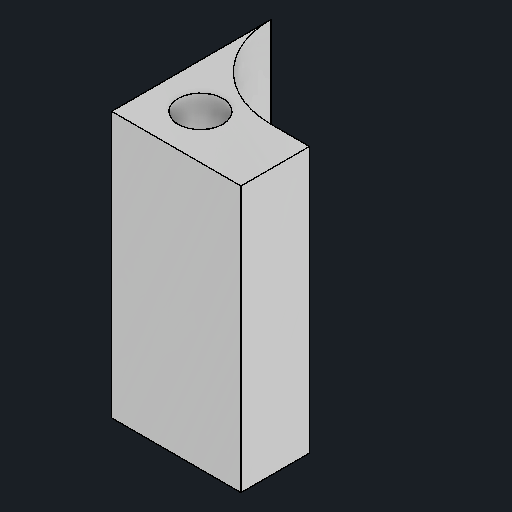
# Autodesk Inventor part: Joint Spacer
Saved by Autodesk Inventor 2026.1 (Build 301233020, 233B)
## iProperties
Created: 2025-05-26
Part Number: Joint Spacer
Material: Aluminum 6061
Document SubType Name: Modeling
Designer: Joshua Eah
Density: 2.7 g/cm^3
Appearance: Machined - Aluminum
Author: Joshua Eah
Autodesk Inventor part; units mm, degrees
ref_plane "YZ Plane" through (0, 0, 0) normal (1, 0, 0) x (0, 1, 0)
ref_plane "XZ Plane" through (0, 0, 0) normal (0, 1, 0) x (-1, 0, 0)
ref_plane "XY Plane" through (0, 0, 0) normal (0, 0, 1) x (1, 0, 0)
sketch "Base" plane through (0, 0, 0) normal (0, 1, 0) x (-1, 0, 0)
  line L0 (0, 0) -> (-12, 0)
  line L1 (-12, 0) -> (-12, -11.4)
  line L2 (-12, -11.4) -> (0, -11.4) construction
  line L3 (0, -11.4) -> (0, 0)
  circle A0 centre (-3.175, -3.175) radius 3.175
  circle A1 centre (-6.5, -11.4) radius 6.5
  line L4 (-6.5, -4.9) -> (-6.5, 0)
  line L5 (-6.5, -4.9) -> (-12, -4.9)
  line L6 (-9.25, -4.9) -> (-9.25, 0)
  point P0 (0, 0)
  point P1 (-12, -7.9359)
  dimension "d24" = 13
  dimension "d21" = 12
  dimension "d22" = 11.4
  dimension "d23" = 6.35
  dimension "d26" = 5.5
  dimension "d36" = 5.5
  constraints: 14 end point, 6 point on line, 3 perpendicular, 2 horizontal, 2 parallel, 2 tangent, 1 centre point, 1 midpoint, 3 other
  measures "d21" distance of L2.end L1.end
  measures "d22" distance of L1.end L0.end
  measures "d23" diameter of A0
  measures "d26" distance from line of L1 point (-6.5, -11.4)
  measures "d36" distance between parallel lines of L1 L4
extrude "Stock" add sketch "Base" against normal blind 19 contours L4 L5 L6 L0 | L0 A0 A1 L4 | L0 L3 A0 | A0 A1 | L3 A1 A0 picked at (-3.3154, -3.7047)
hole "3mm Hole" at (3.175, 0, -3.175) direction (0, -1, 0) diameter 3.2004 end through all clearance for "Socket Head Cap Screw" size "M3" standard "Ansi Metric M Profile"
equation "\"d36\" = d26"
body "Solid2"
